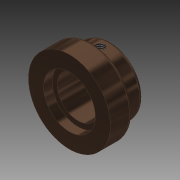
# Autodesk Inventor part: Problem14_15_JacobMorgan_031015_pd3
Saved by Autodesk Inventor 2015 (Build 190159000, 159)
## iProperties
Created: 2015-03-10
Part Number: Problem14_15_JacobMorgan_031015_pd3
Material: Bronze
Document SubType Name: Modeling
Designer: WASHHSST
Density: 8.47 g/cm^3
Appearance: Bronze - Polished
Mass: 89.6487 g
Surface Area: 37.2537 cm^2
Volume: 10.5843 cm^3
Author: WASHHSST
Autodesk Inventor part; units mm, degrees
ref_plane "YZ Plane" through (0, 0, 0) normal (1, 0, 0) x (0, 1, 0)
ref_plane "XZ Plane" through (0, 0, 0) normal (0, 1, 0) x (-1, 0, 0)
sketch "Sketch4" plane through (0, 0, 0) normal (0, 0, 1) x (1, 0, 0)
  circle A0 centre (0, 0) radius 18.923
  dimension "d2" = 37.846
  constraints: 1 centre point, 1 coincident
  measures "d2" diameter of A0
extrude "Extrusion1" add sketch "Sketch4" against normal blind 10.414
sketch "Sketch7" plane through (0, 0, 0) normal (0, 0, 1) x (1, 0, 0)
  circle A0 centre (0, 0) radius 9.525
  dimension "d8" = 19.05
  constraints: 1 centre point, 1 coincident
  measures "d8" diameter of A0
extrude "Extrusion3" cut sketch "Sketch7" against normal blind 127
sketch "Sketch8" plane through (0, 0, 0) normal (0, 0, 1) x (1, 0, 0)
  circle A0 centre (0, 0) radius 11.938
  dimension "d11" = 23.876
  constraints: 1 centre point, 1 coincident
  measures "d11" diameter of A0
extrude "Extrusion4" cut sketch "Sketch8" against normal blind 3.9624
sketch "Sketch9" plane through (0, 0, -10.414) normal (0, 0, -1) x (-1, 0, 0)
  circle A0 centre (0, 0) radius 15.0876
  dimension "d14" = 30.1752
  constraints: 1 centre point, 1 coincident
  measures "d14" diameter of A0
extrude "Extrusion5" add sketch "Sketch9" along normal blind 8.5852
sketch "Sketch10" plane through (0, 0, -10.414) normal (0, 0, 1) x (1, 0, 0)
  circle A0 centre (0, 0) radius 9.525
  constraints: 1 centre point, 1 coincident
extrude "Extrusion6" cut sketch "Sketch10" against normal blind 8.5852
fillet "Fillet1" radius 1.6002 1 edges at (15.0876, 0, -10.414)
fillet "Fillet2" radius 1.6002 1 edges at (-18.923, 0, -10.414)
sketch "Sketch11" plane through (0, 0, -18.9992) normal (0, 0, -1) x (-1, 0, 0)
  circle A0 centre (0, 0) radius 9.525 projected
  line L0 (0, 9.525) -> (0, 15.0876)
  circle A1 centre (0, 0) radius 15.0876 projected
  constraints: 2 end point, 2 vertical alignment, 1 vertical, 2 other
ref_plane "Work Plane2" through (0, 15.0876, -10.414) normal (0, 1, 0) x (-1, 0, 0)
sketch "Sketch12" plane through (0, 15.0876, -10.414) normal (0, 1, 0) x (-1, 0, 0)
  line L0 (0, 10.414) -> (0, -3.8354)
  dimension "d21" = 14.2494
  constraints: 2 end point, 1 vertical
  measures "d21" distance of L0.start L0.end
hole "Hole1" at (0, 15.0876, -14.2494) direction (0, -1, 0) diameter 3.9624 depth 7.2644 thread size "10-32 UNF" class "2B" standard "ANSI Unified Screw Threads"
fillet "Fillet3" radius 1.6002 1 edges at (15.0876, 0, -18.9992)
body "Solid1"
